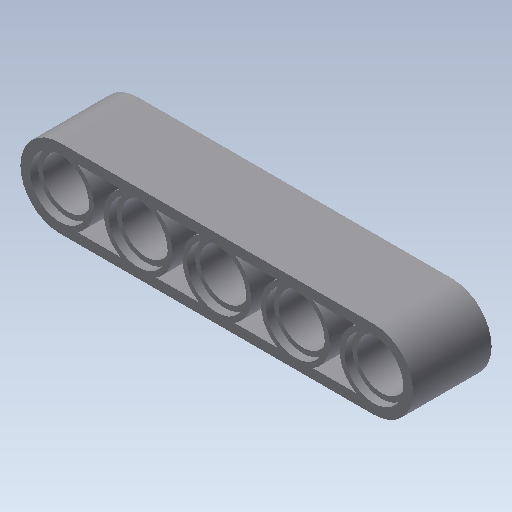
# Autodesk Inventor part: 5M Beam
Saved by Autodesk Inventor 2020 (Build 240168000, 168)
## iProperties
Created: 2014-02-12
Part Number: 5M Beam
Document SubType Name: Modeling
Designer: jleonard
Density: 1 g/cm^3
Material: Generic
Appearance: Default
Author: jleonard
Autodesk Inventor part; units mm, degrees
ref_plane "YZ Plane" through (0, 0, 0) normal (1, 0, 0) x (0, 1, 0)
ref_plane "XZ Plane" through (0, 0, 0) normal (0, 1, 0) x (-1, 0, 0)
ref_plane "XY Plane" through (0, 0, 0) normal (0, 0, 1) x (1, 0, 0)
sketch "Sketch1" plane through (0, 0, 0) normal (0, 0, 1) x (1, 0, 0)
  arc A0 (-16, 4) -> (-16, -4) centre (-16, 0) ccw
  arc A1 (16, -4) -> (16, 4) centre (16, 0) ccw
  line L0 (-16, -4) -> (16, -4)
  line L1 (-16, 4) -> (16, 4)
  line L2 (-28, 0) -> (28, 0) projected
  line L3 (0, -5.6) -> (0, 5.6) projected
  point P0 (0, 0)
  dimension "d3" = 4
  dimension "d4" = 4
  dimension "d5" = 32
  dimension "d6" = 32
  dimension "d7" = 0
  dimension "d8" = 16
  dimension "d9" = 32
  dimension "d10" = 32
  constraints: 4 end point, 4 point on circle, 2 centre point, 2 tangent
  measures "d3" radius of A0
  measures "d4" radius of A1
  measures "d5" distance of L1.start L1.end
  measures "d6" distance of L0.start L0.end
  measures "d7" distance from line of L2 A0.centre
  measures "d8" distance from line of L3 A0.centre
  measures "d9" horizontal distance of A1.centre L0.start
  measures "d10" horizontal distance of A1.centre L1.start
extrude "Extrusion1" add sketch "Sketch1" along normal blind 8
sketch "Sketch2" plane through (0, 0, 8) normal (0, 0, 1) x (1, 0, 0)
  arc A0 (-16, 4) -> (-16, -4) centre (-16, 0) ccw projected
  circle A1 centre (-16, 0) radius 2.5
  line L0 (-28, 0) -> (28, 0) projected
  circle A2 centre (-8, 0) radius 2.5
  circle A3 centre (0, 0) radius 2.5
  circle A4 centre (8, 0) radius 2.5
  circle A5 centre (16, 0) radius 2.5
  dimension "d13" = 5
  dimension "d19" = 8
  constraints: 5 centre point, 1 coincident, 1 horizontal, 8 other
  measures "d13" diameter of A1
  measures "d19" distance of A1.centre A2.centre
extrude "Extrusion2" cut sketch "Sketch2" against normal through all
sketch "Sketch3" plane through (0, 0, 8) normal (0, 0, 1) x (1, 0, 0)
  circle A0 centre (16, 0) radius 2.5 projected
  circle A1 centre (8, 0) radius 2.5 projected
  circle A2 centre (0, 0) radius 2.5 projected
  circle A3 centre (-8, 0) radius 2.5 projected
  circle A4 centre (-16, 0) radius 2.5 projected
  arc A5 (-16, 4) -> (-16, -4) centre (-16, 0) ccw projected
  circle A6 centre (-16, 0) radius 3
  line L0 (-28, 0) -> (28, 0) projected
  circle A7 centre (-8, 0) radius 3
  circle A8 centre (0, 0) radius 3
  circle A9 centre (8, 0) radius 3
  circle A10 centre (16, 0) radius 3
  dimension "d23" = 6
  dimension "d29" = 8
  constraints: 5 centre point, 1 coincident, 1 horizontal, 8 other
  measures "d23" diameter of A6
  measures "d29" distance of A6.centre A7.centre
extrude "Extrusion3" cut sketch "Sketch3" against normal blind 0.8 contours L0 A10 A0 | A0 L0 A10 | A6 L0 A4 | L0 A4 A6 | A7 L0 A3 | L0 A3 A7 | A8 L0 A2 | L0 A2 A8 | A9 L0 A1 | L0 A1 A9
sketch "Sketch4" plane through (0, 0, 0) normal (0, 0, -1) x (-1, 0, 0)
  circle A0 centre (-16, 0) radius 2.5 projected
  circle A1 centre (-8, 0) radius 2.5 projected
  circle A2 centre (0, 0) radius 2.5 projected
  circle A3 centre (8, 0) radius 2.5 projected
  circle A4 centre (16, 0) radius 2.5 projected
  arc A5 (-16, 4) -> (-16, -4) centre (-16, 0) ccw projected
  circle A6 centre (-16, 0) radius 3
  line L0 (28, 0) -> (-28, 0) projected
  circle A7 centre (-8, 0) radius 3
  circle A8 centre (0, 0) radius 3
  circle A9 centre (8, 0) radius 3
  circle A10 centre (16, 0) radius 3
  dimension "d33" = 6
  dimension "d39" = 8
  constraints: 5 centre point, 1 coincident, 1 horizontal, 8 other
  measures "d33" diameter of A6
  measures "d39" distance of A6.centre A7.centre
extrude "Extrusion4" cut sketch "Sketch4" against normal blind 0.8 contours L0 A6 A0 | A0 L0 A6 | A10 L0 A4 | L0 A4 A10 | A9 L0 A3 | L0 A3 A9 | A8 L0 A2 | L0 A2 A8 | A7 L0 A1 | L0 A1 A7
sketch "Sketch5" plane through (0, 0, 8) normal (0, 0, 1) x (1, 0, 0)
  circle A0 centre (-8, 0) radius 3 projected
  arc A1 (-16, 4) -> (-16, -4) centre (-16, 0) ccw projected
  arc A2 (-14.1972, -3) -> (-14.1972, 3) centre (-16, 0) ccw
  arc A3 (-9.8028, 3) -> (-9.8028, -3) centre (-8, 0) ccw
  line L0 (-14.1972, 3) -> (-9.8028, 3)
  line L1 (-14.1972, -3) -> (-9.8028, -3)
  line L2 (-28, 0) -> (28, 0) projected
  arc A4 (-6.1972, -3) -> (-6.1972, 3) centre (-8, 0) ccw
  arc A5 (-1.8028, 3) -> (-1.8028, -3) centre (0, 0) ccw
  line L3 (-6.1972, 3) -> (-1.8028, 3)
  line L4 (-6.1972, -3) -> (-1.8028, -3)
  arc A6 (1.8028, -3) -> (1.8028, 3) centre (0, 0) ccw
  arc A7 (6.1972, 3) -> (6.1972, -3) centre (8, 0) ccw
  line L5 (1.8028, 3) -> (6.1972, 3)
  line L6 (1.8028, -3) -> (6.1972, -3)
  arc A8 (9.8028, -3) -> (9.8028, 3) centre (8, 0) ccw
  arc A9 (14.1972, 3) -> (14.1972, -3) centre (16, 0) ccw
  line L7 (9.8028, 3) -> (14.1972, 3)
  line L8 (9.8028, -3) -> (14.1972, -3)
  dimension "d43" = 3.5
  dimension "d44" = 3.5
  dimension "d45" = 4.3944
  dimension "d46" = 4.3944
  dimension "d52" = 8
  constraints: 16 end point, 16 point on circle, 8 centre point, 2 coincident, 2 tangent, 1 horizontal, 30 other
  measures "d43" radius of A2
  measures "d44" radius of A3
  measures "d45" distance of L0.start L0.end
  measures "d46" distance of L1.start L1.end
  measures "d52" distance of L0.start L3.start
extrude "Extrusion5" cut sketch "Sketch5" against normal through all contours A3 L1 A2 L2 | L2 A2 L0 A3 | A8 L7 A9 L2 | L2 A9 L8 A8 | A6 L5 A7 L2 | L2 A7 L6 A6 | A4 L3 A5 L2 | L2 A5 L4 A4
body "Solid1"
